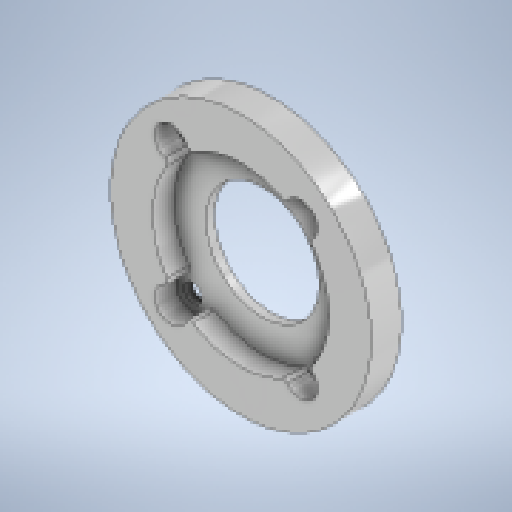
# Autodesk Inventor part: frame_motor_support_top
Saved by Autodesk Inventor 2026.1 (Build 301233000, 233)
## iProperties
Created: 2023-10-02
Part Number: frame_motor_support_top
Material: Aluminum 6061-AHC
Document SubType Name: Modeling
Designer: chanh
Density: 2.7 g/cm^3
Appearance: Aluminum - Dark
Author: chanh
Autodesk Inventor part; units mm, degrees
ref_plane "YZ Plane" through (0, 0, 0) normal (1, 0, 0) x (0, 1, 0)
ref_plane "XZ Plane" through (0, 0, 0) normal (0, 1, 0) x (-1, 0, 0)
ref_plane "XY Plane" through (0, 0, 0) normal (0, 0, 1) x (1, 0, 0)
sketch "Sketch8" plane through (0, 0, 0) normal (0, 0, 1) x (1, 0, 0)
  circle A0 centre (0, 0) radius 15
  dimension "d33" = 30
  constraints: 1 centre point, 1 coincident
  measures "d33" diameter of A0
extrude "Extrusion7" add sketch "Sketch8" against normal blind 8
sketch "Sketch10" plane through (0, 0, -8) normal (0, 0, -1) x (-1, 0, 0)
  line L0 (9, 10.07) -> (-29.1, 10.07)
  arc A0 (10, 9.07) -> (9, 10.07) centre (9, 9.07) ccw
  line L1 (10, 9.07) -> (10, -9.07)
  arc A1 (9, -10.07) -> (10, -9.07) centre (9, -9.07) ccw
  line L2 (-29.1, -10.07) -> (9, -10.07)
  line L3 (-29.1, 10.07) -> (-29.1, -10.07)
  line L4 (10.4, -9.07) -> (10.4, 9.07)
  arc A2 (10.4, 9.07) -> (9, 10.47) centre (9, 9.07) ccw
  line L5 (9, 10.47) -> (-29.5, 10.47)
  line L6 (-29.5, 10.47) -> (-29.5, -10.47)
  line L7 (-29.5, -10.47) -> (9, -10.47)
  arc A3 (9, -10.47) -> (10.4, -9.07) centre (9, -9.07) ccw
  dimension "d59" = 0.4
  constraints: 16 end point, 8 point on circle, 4 centre point, 2 horizontal, 2 vertical, 15 other
  measures "d59" distance between parallel lines of L1 L4
extrude "Extrusion8" cut sketch "Sketch10" against normal blind 2 contours A0 L1 A1 L2 L3 L0 | A3 L7 L6 L5 A2 L4
sketch "Sketch11" plane through (0, 0, -6) normal (0, 0, -1) x (-1, 0, 0)
  circle A0 centre (0, 0) radius 6.4
  circle A1 centre (0, 0) radius 6.5
  point P0 (0, 0)
  dimension "d58" = 13
  constraints: 2 centre point, 1 coincident, 2 other
  measures "d58" diameter of A1
extrude "Extrusion9" cut sketch "Sketch11" against normal through all contours A0 | A1
sketch "Sketch13" plane through (0, 0, 0) normal (0, 0, 1) x (1, 0, 0)
  circle A0 centre (0, 0) radius 9.96
  circle A1 centre (0, 0) radius 10.16
  point P0 (0, 0)
  dimension "d44" = 0.2
  constraints: 2 centre point, 2 other
  measures "d44" radial gap between concentric circles of A0 A1
extrude "Extrusion11" cut sketch "Sketch13" against normal blind 3 contours A0 | A1
sketch "Sketch14" plane through (0, 0, 0) normal (0, 0, 1) x (1, 0, 0)
  circle A0 centre (6.9, 8) radius 0.7835
  circle A1 centre (6.9, -8) radius 0.7835
  circle A2 centre (-8, 8.07) radius 1
  circle A3 centre (-8, -8.07) radius 1
  point P0 (0, 0)
  constraints: 4 centre point, 8 other
hole "Hole2" at (6.9, 8, 0) at (-8, 8.07, 0) at (-8, -8.07, 0) at (6.9, -8, 0) direction (0, 0, -1) diameter 2.1 end through all
sketch "Sketch15" plane through (0, 0, 0) normal (0, 0, 1) x (1, 0, 0)
  arc A0 (7.3255, 7.0401) -> (5.888, 8.2799) centre (6.9, 8) ccw projected
  arc A1 (5.888, -8.2799) -> (7.3255, -7.0401) centre (6.9, -8) ccw projected
  circle A2 centre (-8, 8.07) radius 1.05 projected
  circle A3 centre (-8, -8.07) radius 1.05 projected
  circle A4 centre (6.9, 8) radius 1.9
  circle A5 centre (6.9, -8) radius 1.9
  circle A6 centre (-8, -8.07) radius 1.9
  circle A7 centre (-8, 8.07) radius 1.9
  point P0 (0, 0)
  dimension "d54" = 3.8
  constraints: 4 centre point, 4 coincident, 3 equal radius
  measures "d54" diameter of A4
extrude "Extrusion12" cut sketch "Sketch15" against normal blind 4.5 contours A2 | A3 | A4 | A5 | A6 | A7
fillet "Fillet2" radius 0.5 8 edges at (5.1562, 8.7544, -1.5) (7.9023, 6.3859, -1.5) (-6.1008, 8.1244, -1.5) (-8.071, 6.1713, -1.5) (-8.071, -6.1713, -1.5) (-6.1008, -8.1244, -1.5) (5.1562, -8.7544, -1.5) (7.9023, -6.3859, -1.5)
sketch "Sketch16" plane through (0, 0, -8) normal (0, 0, -1) x (-1, 0, 0)
  circle A0 centre (-6.9, -8) radius 1.05 projected
  circle A1 centre (8, -8.07) radius 1.05 projected
  circle A2 centre (8, 8.07) radius 1.05 projected
  circle A3 centre (-6.9, 8) radius 1.05 projected
  circle A4 centre (0, 0) radius 6.5 projected
  arc A5 (-10.7415, 10.47) -> (-10.7415, -10.47) centre (0, 0) ccw projected
  line L0 (9, -10.47) -> (-10.7415, -10.47) projected
  arc A6 (9, -10.47) -> (10.4, -9.07) centre (9, -9.07) ccw projected
  line L1 (10.4, 9.07) -> (10.4, -9.07) projected
  arc A7 (10.4, 9.07) -> (9, 10.47) centre (9, 9.07) ccw projected
  line L2 (-10.7415, 10.47) -> (9, 10.47) projected
  line L3 (-10.7415, 10.47) -> (9, 10.47) projected
  arc A8 (10.4, 9.07) -> (9, 10.47) centre (9, 9.07) ccw projected
  line L4 (10.4, 9.07) -> (10.4, -9.07) projected
  arc A9 (9, -10.47) -> (10.4, -9.07) centre (9, -9.07) ccw projected
  line L5 (9, -10.47) -> (-10.7415, -10.47) projected
  arc A10 (-10.7415, -10.47) -> (-10.7415, 10.47) centre (0, 0) ccw projected
sketch "Sketch17" plane through (0, 0, -3) normal (0, 0, 1) x (1, 0, 0)
  circle A0 centre (6.9, 8) radius 1.05 projected
  circle A1 centre (6.9, 8) radius 1.9 projected
  circle A2 centre (6.9, -8) radius 1.05 projected
  circle A3 centre (6.9, -8) radius 1.9 projected
  circle A4 centre (-8, 8.07) radius 1.05 projected
  circle A5 centre (-8, 8.07) radius 1.9 projected
  circle A6 centre (-8, -8.07) radius 1.05 projected
  circle A7 centre (-8, -8.07) radius 1.9 projected
  point P0 (0, 0)
extrude "Extrusion13" add sketch "Sketch17" against normal blind 1.5
extrude "Extrusion14" cut sketch "Sketch16" against normal blind 3.5
sketch "Sketch18" plane through (0, 0, -3) normal (0, 0, 1) x (1, 0, 0)
  circle A0 centre (-8, 8.07) radius 1.05 projected
  circle A1 centre (6.9, -8) radius 1.05 projected
  circle A2 centre (-8, -8.07) radius 1.05 projected
  circle A3 centre (6.9, 8) radius 1.05 projected
  arc A4 (-8.4935, 5.5754) -> (-8.7216, 6.3124) centre (-8.9115, 5.8498) ccw projected
  arc A5 (-8.4935, 5.5754) -> (-8.4935, -5.5754) centre (0, 0) ccw projected
  arc A6 (-8.7216, -6.3124) -> (-8.4935, -5.5754) centre (-8.9115, -5.8498) ccw projected
  arc A7 (-8.7216, -6.3124) -> (-6.2361, -8.7763) centre (-8, -8.07) ccw projected
  arc A8 (-5.5012, -8.5418) -> (-6.2361, -8.7763) centre (-5.772, -8.9621) ccw projected
  arc A9 (-5.5012, -8.5418) -> (4.7389, -8.9871) centre (0, 0) ccw projected
  arc A10 (5.3737, -9.1316) -> (4.7389, -8.9871) centre (4.9721, -9.4294) ccw projected
  arc A11 (5.3737, -9.1316) -> (8.2435, -6.6565) centre (6.9, -8) ccw projected
  arc A12 (8.1938, -6.0073) -> (8.2435, -6.6565) centre (8.597, -6.3029) ccw projected
  arc A13 (8.1938, -6.0073) -> (8.1938, 6.0073) centre (0, 0) ccw projected
  arc A14 (8.2435, 6.6565) -> (8.1938, 6.0073) centre (8.597, 6.3029) ccw projected
  arc A15 (8.2435, 6.6565) -> (5.3737, 9.1316) centre (6.9, 8) ccw projected
  arc A16 (4.7389, 8.9871) -> (5.3737, 9.1316) centre (4.9721, 9.4294) ccw projected
  arc A17 (4.7389, 8.9871) -> (-5.5012, 8.5418) centre (0, 0) ccw projected
  arc A18 (-6.2361, 8.7763) -> (-5.5012, 8.5418) centre (-5.772, 8.9621) ccw projected
  arc A19 (-6.2361, 8.7763) -> (-8.7216, 6.3124) centre (-8, 8.07) ccw projected
  circle A20 centre (0, 0) radius 6.5 projected
  point P0 (0, 0)
extrude "Extrusion15" cut sketch "Sketch18" against normal blind 0.5
sketch "Sketch19" plane through (0, 0, 0) normal (0, 0, 1) x (1, 0, 0)
  circle A0 centre (0, 0) radius 15 projected
  arc A1 (8.1938, -6.0073) -> (8.2435, -6.6565) centre (8.597, -6.3029) ccw projected
  arc A2 (5.3737, -9.1316) -> (8.2435, -6.6565) centre (6.9, -8) ccw projected
  arc A3 (5.3737, -9.1316) -> (4.7389, -8.9871) centre (4.9721, -9.4294) ccw projected
  arc A4 (-5.5012, -8.5418) -> (4.7389, -8.9871) centre (0, 0) ccw projected
  arc A5 (-5.5012, -8.5418) -> (-6.2361, -8.7763) centre (-5.772, -8.9621) ccw projected
  arc A6 (-8.7216, -6.3124) -> (-6.2361, -8.7763) centre (-8, -8.07) ccw projected
  arc A7 (-8.7216, -6.3124) -> (-8.4935, -5.5754) centre (-8.9115, -5.8498) ccw projected
  arc A8 (-8.4935, 5.5754) -> (-8.4935, -5.5754) centre (0, 0) ccw projected
  arc A9 (-8.4935, 5.5754) -> (-8.7216, 6.3124) centre (-8.9115, 5.8498) ccw projected
  arc A10 (-6.2361, 8.7763) -> (-8.7216, 6.3124) centre (-8, 8.07) ccw projected
  arc A11 (-6.2361, 8.7763) -> (-5.5012, 8.5418) centre (-5.772, 8.9621) ccw projected
  arc A12 (4.7389, 8.9871) -> (-5.5012, 8.5418) centre (0, 0) ccw projected
  arc A13 (4.7389, 8.9871) -> (5.3737, 9.1316) centre (4.9721, 9.4294) ccw projected
  arc A14 (8.2435, 6.6565) -> (5.3737, 9.1316) centre (6.9, 8) ccw projected
  arc A15 (8.2435, 6.6565) -> (8.1938, 6.0073) centre (8.597, 6.3029) ccw projected
  arc A16 (8.1938, -6.0073) -> (8.1938, 6.0073) centre (0, 0) ccw projected
extrude "Extrusion16" cut sketch "Sketch19" against normal blind 1
body "Solid2"
